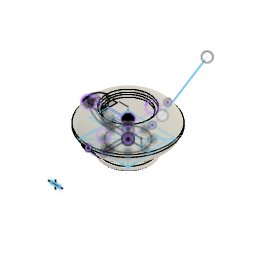
Pin_50% v4 (Autodesk Fusion 360 design; units mm, degrees)
Autodesk Fusion 360 part; units mm, degrees
note: some values were not read from the file. Set by a fixed rule: which sketch regions a step uses.
sketch "Esquisse1" plane through (0, 0, 0) normal (0, 1, 0) x (1, 0, 0)
  line L0 (0, 0) -> (-20, 0)
  line L1 (0, 0) -> (0, -4)
  line L2 (0, 0) -> (0, -10) construction
  line L3 (0, -10) -> (-32.5, -10)
  line L4 (-32.5, -10) -> (-29.5, -10)
  arc A0 (-20, 0) -> (-32.5, -10) centre (-20, -12.8125) ccw
  line L5 (0, -4) -> (-20, -4)
  line L6 (-29.5, -10) -> (-29.5, -7.9)
  line L7 (-29.5, -7.9) -> (-26.5, -7.9)
  arc A1 (-20, -4) -> (-26.5, -7.9) centre (-20, -11.3667) ccw
  dimension "d1" = 20
  dimension "d2" = 4
  dimension "d6" = 10
  dimension "d7" = 32.5
  dimension "d8" = 3
  dimension "d9" = 2.1
  dimension "d10" = 3
  dimension "d11" = 20
  constraint coincident L0.start L1.start
  constraint horizontal L0
  constraint perpendicular L0 L1
  constraint perpendicular L0 L2
  constraint perpendicular L2 L3
  constraint parallel L3 L4
  constraint tangent L0 A0
  constraint perpendicular L2 L5
  constraint perpendicular L3 L6
  constraint perpendicular L6 L7
  constraint tangent L5 A1
  measures "d1" distance of L0.start L0.end
  measures "d2" distance of L0.start L1.end
  measures "d6" distance of L0.start L2.end
  measures "d7" distance of L2.end L3.end
  measures "d8" distance of L3.end L4.end
  measures "d9" distance of L4.end L6.end
  measures "d10" distance of L6.end L7.end
  measures "d11" distance of L1.end L5.end
sketch "Esquisse4" plane through (0, 0, 0) normal (0, 1, 0) x (1, 0, 0)
  line L0 (-32.5, -10) -> (-32.5, -12)
  line L1 (-32.5, -12) -> (-28.35, -12)
  line L2 (-28.35, -12) -> (-28.35, -14)
  line L3 (-28.35, -14) -> (0, -14)
  line L4 (0, -14) -> (0, -8)
  line L5 (-32.5, -10) -> (-29.35, -10)
  line L6 (-29.35, -10) -> (-29.35, -8)
  line L7 (-29.35, -8) -> (0, -8)
  point P0 (-32.5, -10)
  point P1 (0, -4)
  dimension "d19" = 2
  dimension "d20" = 2
  dimension "d25" = 4.15
  dimension "d26" = 2
  dimension "d32" = 3.15
  constraint perpendicular L0 L1
  constraint perpendicular L1 L2
  constraint perpendicular L2 L3
  constraint perpendicular L3 L4
  constraint perpendicular L0 L5
  constraint perpendicular L5 L6
  constraint perpendicular L4 L7
  constraint coincident P0 L0.start
  constraint horizontal L7
  constraint vertical L4.end P1
  measures "d19" distance of P0 L0.end
  measures "d20" distance of L1.end L2.end
  measures "d25" distance of L0.end L1.end
  measures "d26" distance of L5.end L6.end
  measures "d32" distance of P0 L5.end
sketch "Esquisse6" plane through (0, 0, 0) normal (0, 1, 0) x (1, 0, 0)
  line L0 (0, -14) -> (0, -23) construction
  line L1 (0, -23) -> (-17.65, -23) construction
  line L2 (-32.5, -12) -> (-30.5, -12)
  arc A0 (-32.5, -12) -> (-17.65, -23) centre (-15.1932, -4.1595) ccw
  line L3 (-17.65, -23) -> (-17.65, -20.75)
  line L4 (-30.5, -12) -> (-28.5, -12)
  line L5 (-28.5, -14.1) -> (-26.5, -14.1)
  line L6 (-26.5, -14.1) -> (-26.5, -15.85)
  line L7 (-28.5, -12) -> (-28.5, -14.1)
  line L8 (-17.65, -20.75) -> (-15.65, -20.75)
  line L9 (-15.65, -20.75) -> (-15.65, -18.75)
  line L10 (-15.65, -18.75) -> (-17.9, -18.75)
  arc A1 (-26.5, -15.85) -> (-17.9, -18.75) centre (-17.9, -4.5483) ccw
  line L11 (-28.35, -12) -> (-28.35, -14)
  line L12 (-28.35, -14) -> (0, -14)
  point P0 (-32.5, -10)
  point P1 (0, -14)
  dimension "d27" = 9
  dimension "d28" = 17.65
  dimension "d69" = 2.1
  dimension "d70" = 1.75
  dimension "d71" = 2.25
  dimension "d72" = 2
  dimension "d73" = 2
  dimension "d74" = 2.25
  dimension "d99" = 0.15
  dimension "d100" = 0.1
  dimension "d101" = 2
  dimension "d102" = 19
  constraint vertical L0
  constraint perpendicular L0 L1
  constraint parallel L1 L2
  constraint perpendicular L1 L3
  constraint parallel L2 L4
  constraint perpendicular L5 L6
  constraint perpendicular L5 L7
  constraint perpendicular L3 L8
  constraint perpendicular L8 L9
  constraint perpendicular L9 L10
  constraint vertical L2.start P0
  constraint coincident L0.start L12.end
  constraint tangent L10 A1
  measures "d27" distance of L0.start L0.end
  measures "d28" distance of L0.end L1.end
  measures "d69" distance of L4.end L5.start
  measures "d70" distance of L5.end L6.end
  measures "d71" distance of L1.end L3.end
  measures "d72" distance of L3.end L8.end
  measures "d73" distance of L8.end L9.end
  measures "d74" distance of L9.end L10.end
  measures "d99" distance of L7 L11
  measures "d100" distance of L5 L12
  measures "d101" distance of L5.start L5.end
  measures "d102" radius of A0
revolve "Révolution1" add sketch "Esquisse1" angle 360 about axis through (0, 0, 0) along (0, 0, 1) makes body 1
revolve "Révolution2" add sketch "Esquisse4" angle 360 about axis through (0, 0, 14) along (0, 0, -1) separate body makes body 2
revolve "Révolution3" add sketch "Esquisse6" angle 360 about axis through (0, 0, 14) along (0, 0, 1) separate body makes body 3
sketch "Esquisse7" plane through (0, 0, 0) normal (0, 0, -1) x (1, 0, 0)
  circle A0 centre (0, 0) radius 10
  line L0 (-20, 20) -> (20, 20)
  line L1 (20, 20) -> (20, -20)
  line L2 (20, -20) -> (-20, -20)
  line L3 (-20, -20) -> (-20, 20)
  line L4 (-20, 20) -> (20, -20)
  line L5 (20, 20) -> (-20, -20)
  line L6 (-20, 20) -> (-20, 7.5)
  line L7 (-20, -20) -> (-20, -7.5)
  line L8 (0, -20) -> (0, 20)
  line L9 (20, 0) -> (-20, 0)
  circle A1 centre (0, 0) radius 13.75
  point P0 (9.7227, -9.7227)
  point P1 (0, -13.75)
  point P2 (-9.7227, -9.7227)
  point P3 (13.75, 0)
  point P4 (-13.75, 0)
  point P5 (-9.7227, 9.7227)
  point P6 (0, 13.75)
  point P7 (9.7227, 9.7227)
  dimension "d33" = 80
  dimension "d34" = 80
  dimension "d35" = 25
  dimension "d36" = 25
  dimension "d104" = 55
  constraint horizontal L0
  constraint vertical L1
  constraint horizontal L2
  constraint vertical L3
  constraint coincident L3 L6.end
  constraint coincident L3 L7.end
  constraint midpoint L2 L8.start
  constraint midpoint L0 L8.end
  constraint midpoint L1 L9.start
  constraint midpoint L3 L9.end
  constraint coincident A0.centre A1.centre
  constraint coincident L4 P0
  constraint coincident A1 P0
  constraint coincident A1 P1
  constraint coincident L8 P1
  constraint coincident L5 P2
  constraint coincident A1 P2
  constraint coincident L9 P3
  constraint coincident A1 P3
  constraint coincident L9 P4
  constraint coincident A1 P4
  constraint coincident L4 P5
  constraint coincident A1 P5
  constraint coincident L8 P6
  constraint coincident A1 P6
  constraint coincident L5 P7
  constraint coincident A1 P7
sketch "Esquisse8" plane through (0, 0, 0) normal (1, 0, 0) x (0, 1, 0)
  line L0 (0, 0) -> (-17.5, 0)
  line L1 (0, 0) -> (0, 3)
  line L2 (0, 3) -> (-17.5, 3)
  arc A0 (-17.5, 3) -> (-17.5, 0) centre (-17.5, 1.5) ccw
  dimension "d49" = 17.5
  dimension "d50" = 17.5
  dimension "d52" = 3
  constraint coincident L0.start L1.start
  constraint horizontal L0
  constraint perpendicular L0 L1
  constraint perpendicular L1 L2
  constraint tangent L2 A0
  measures "d49" distance of L0.start L0.end
  measures "d50" distance of L1.end L2.end
  measures "d52" distance of L0.start L1.end
revolve "Révolution4" add sketch "Esquisse8" angle 360 about axis through (0, 0, 1.75) along (0, 0, 1) separate body makes body 4
sketch "Esquisse9" plane through (0, 0, 0) normal (1, 0, 0) x (0, 1, 0)
  line L0 (64.9747, 25.8669) -> (28.0897, 2.7613)
  line L1 (0, 10) -> (32.5, 10)
  line L2 (-32.5, 10) -> (0, 10)
  line L3 (0, 0) -> (20, 0)
  line L4 (-20, 0) -> (0, 0)
  arc A0 (20, 0) -> (32.5, 10) centre (20, 12.8125) ccw
  arc A1 (-32.5, 10) -> (-20, 0) centre (-20, 12.8125) ccw
  constraint tangent L0 A0
ref_plane "Plan de construction1" through (0, 46.5322, 14.3141) normal (0, -0.530866, 0.847456) x (0, -0.847456, -0.530866)
move_body "Déplacer4" bodies 4 to x (1, 0, 0) y (0, 1, 0) z (0, 0, 1) at (0, 0, -25)
sketch "Esquisse10" plane through (0, 0, 0) normal (0, 1, 0) x (1, 0, 0)
  line L0 (0, 0) -> (11, 0)
  line L1 (11, 0) -> (11, -6)
  line L2 (11, -6) -> (0, -6)
  line L3 (0, -6) -> (0, 0)
  dimension "d135" = 11
  dimension "d136" = 6
  constraint horizontal L0
  constraint vertical L1
  constraint horizontal L2
  constraint vertical L3
  constraint coincident L0.start L3.end
  measures "d135" distance of L0.start L0.end
  measures "d136" distance of L0.start L2.end
extrude "Extrusion1" add sketch "Esquisse10" against normal blind 9 separate body makes body 5
move_body "Déplacer5" bodies 5 to x (1, 0, 0) y (0, 1, 0) z (0, 0, 1) at (0, -56, 0)
sketch "Esquisse11" plane through (0, -65, 0) normal (0, -1, 0) x (1, 0, 0)
  line L0 (11, 6) -> (0, 6)
  line L1 (0, 6) -> (0, 0)
  line L2 (0, 0) -> (11, 0)
  line L3 (11, 0) -> (11, 6)
  line L4 (5.5, 6) -> (5.5, 0)
  line L5 (0, 3) -> (11, 3)
  line L6 (1.9733, 3.9895) -> (9.0733, 3.9895)
  line L7 (9.0733, 3.9895) -> (9.0733, 1.9895)
  line L8 (9.0733, 1.9895) -> (1.9733, 1.9895)
  line L9 (1.9733, 1.9895) -> (1.9733, 3.9895)
  dimension "d139" = 7.1
  dimension "d140" = 2
  constraint midpoint L0 L4.start
  constraint midpoint L2 L4.end
  constraint midpoint L1 L5.start
  constraint midpoint L3 L5.end
  constraint horizontal L6
  constraint vertical L7
  constraint horizontal L8
  constraint vertical L9
  measures "d139" distance of L6.start L6.end
  measures "d140" distance of L6.start L8.end
extrude "Extrusion2" add sketch "Esquisse11" along normal blind 6 contours L4 L5 L6 L7 | L4 L5 L6 L9 | L4 L5 L7 L8 | L4 L5 L8 L9 bodies 5
move_body "Déplacer6" bodies 5 to x (-1, 0, 0) y (0, -1, 0) z (0, 0, 1) at (0, -142, 0)
move_body "Déplacer7" bodies 5 to x (1, 0, 0) y (0, 1, 0) z (0, 0, 1) at (6, 23, 6)
combine "Combiner1" operation cut target body 1 tool bodies 5
sketch "Esquisse12" plane through (0, 0, 7) normal (0, 0, 1) x (1, 0, 0)
  line L0 (24, -7.5) -> (16.5, -7.5)
  line L1 (16.5, -7.5) -> (16.5, 7.5)
  line L2 (16.5, 7.5) -> (24, 7.5)
  line L3 (24, 7.5) -> (24, -7.5)
  line L4 (0, 0) -> (16.5, 0) construction
  line L5 (0, 0) -> (-16.5, 0)
  line L6 (-16.3059, 0) -> (-16.3059, 7.5)
  line L7 (-16.3059, 7.5) -> (-23.8059, 7.5)
  line L8 (-23.8059, 7.5) -> (-23.8059, -7.5)
  line L9 (-23.8059, -7.5) -> (-16.3059, -7.5)
  line L10 (-16.3059, -7.5) -> (-16.3059, 0)
  dimension "d143" = 15
  dimension "d144" = 30
  dimension "d145" = 33
  dimension "d146" = 33
  dimension "d147" = 15
  dimension "d148" = 15
  dimension "d149" = 30
  dimension "d150" = 15
  dimension "d151" = 15
  constraint horizontal L0
  constraint vertical L1
  constraint horizontal L2
  constraint vertical L3
  constraint coincident L4.start L5.start
  constraint midpoint L1 L4.end
  constraint parallel L4 L5
  constraint coincident L5 L6.start
  constraint perpendicular L5 L6
  constraint perpendicular L1 L7
  constraint perpendicular L5 L8
  constraint perpendicular L1 L9
  constraint coincident L6 L10.end
scale "Echelle1" [no effect]
extrude "Extrusion4" add sketch "Esquisse12" along normal blind 10 separate body makes body 6 at (-16.3059, -2.5, 10.3333) makes body 7 at (16.5, -2.5, 10.3333)
combine "Combiner4" operation cut target body 2 tool bodies 7 6
scale "Echelle2" [no effect]
hole "Perçage27" at (0, -13.75, 0) at (13.75, 0, 0) at (0, 13.75, 0) at (-13.75, 0, 0) at (0, 0, 0) direction (0, 0, 1) diameter 5.15 depth 2.3 tip angle 180 bodies 1
move_body "Déplacer9" bodies 4 to x (1, 0, 0) y (0, 1, 0) z (0, 0, 1) at (0, 0, 25)
hole "Perçage28" at (0, -13.75, 0) at (-13.75, 0, 0) at (0, 13.75, 0) at (13.75, 0, 0) at (0, 0, 0) direction (0, 0, 1) diameter 5.15 depth 2.3 tip angle 180 bodies 4
extrude "Extrusion5" add sketch "Esquisse11" against normal blind 5 separate body makes body 8
extrude "Extrusion6" add sketch "Esquisse11" along normal blind 4 contours L4 L5 L6 L7 | L4 L5 L6 L9 | L4 L5 L7 L8 | L4 L5 L8 L9 bodies 8
move_body "Déplacer10" bodies 8 to x (-1, 0, 0) y (0, -1, 0) z (0, 0, 1) at (5, -105, 3)
extrude "Extrusion7" add 1 faces at (-1.7066, -37.3333, 6.9895) along direction (0, 0, 1) blind 1 on bodies 8 bodies 8
extrude "Extrusion8" add 1 faces at (-1.7066, -37.3333, 4.9895) along direction (0, 0, -1) blind 1 on bodies 8 bodies 8
extrude "Extrusion9" add 1 faces at (1.3333, -45, 7) along direction (0, -1, 0) blind 1 on bodies 8 bodies 8
extrude "Extrusion10" add 1 faces at (1.3333, -46, 7) along direction (0, -1, 0) blind 2 on bodies 8 bodies 8
move_body "Déplacer11" bodies 8 to x (1, 0, 0) y (0, 1, 0) z (0, 0, 1) at (0, 15, 0)
move_body "Déplacer12" bodies 8 to x (1, 0, 0) y (0, 1, 0) z (0, 0, 1) at (0, 0, -1)
move_body "Déplacer13" bodies 8 to x (-1, 0, 0) y (0, -1, 0) z (0, 0, 1) at (-12, -85, 0)
move_face "DéplacerFace1" by (0, 10, 0) 1 faces at (-13.3333, -52, 6) on bodies 8
move_body "Déplacer14" bodies 8 to x (1, 0, 0) y (0, 1, 0) z (0, 0, 1) at (10, 25, 0)
combine "Combiner5" operation cut target body 1 tool bodies 8
move_body "Déplacer15" bodies 4 to x (1, 0, 0) y (0, 1, 0) z (0, 0, 1) at (0, 0, -10)
equation "d1 = 40 * Echelle"
equation "d6 = 20 * Echelle"
equation "d7 = 65 * Echelle"
equation "d11 = 40 * Echelle"
equation "d27 = 18 * Echelle"
equation "d49 = 35 * Echelle"
equation "d50 = 35 * Echelle"
equation "d70 = 3.5 * Echelle"
equation "d71 = 4.5 * Echelle"
equation "d74 = 4.5000 * Echelle"
equation "d102 = 38 * Echelle"
equation "Echelle = 0.5 mm"
